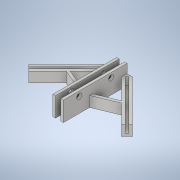
# Autodesk Inventor part: coffee
Saved by Autodesk Inventor 2021.1 (Build 251245010, 245A)
## iProperties
Created: 2019-12-05
Part Number: coffee
Material: Generic
Document SubType Name: Modeling
Designer: Christian
Density: 1 g/cm^3
Appearance: Default
Author: Christian
Autodesk Inventor part; units mm, degrees
ref_plane "YZ Plane" through (0, 0, 0) normal (1, 0, 0) x (0, 1, 0)
ref_plane "XZ Plane" through (0, 0, 0) normal (0, 1, 0) x (-1, 0, 0)
ref_plane "XY Plane" through (0, 0, 0) normal (0, 0, 1) x (1, 0, 0)
sketch "support_base" plane through (0, 0, 0) normal (0, 0, 1) x (1, 0, 0)
  line L0 (-24.7251, -5.2251) -> (20.2749, -5.2251)
  line L1 (20.2749, -5.2251) -> (20.2749, 0.7749)
  line L2 (20.2749, 0.7749) -> (-24.7251, 0.7749)
  line L3 (-24.7251, 0.7749) -> (-24.7251, -5.2251)
  line L4 (-24.7251, -5.2251) -> (20.2749, 0.7749) construction
  line L5 (20.2749, -5.2251) -> (-24.7251, 0.7749) construction
  line L6 (20.2749, 0.7749) -> (-11.5449, 32.5947)
  line L7 (-11.5449, 32.5947) -> (-10.1307, 34.009)
  line L8 (-10.1307, 34.009) -> (21.6892, 2.1892)
  line L9 (21.6892, 2.1892) -> (20.2749, 0.7749)
  line L10 (21.6892, 2.1892) -> (24.6892, -0.8108)
  line L11 (24.6892, -0.8108) -> (20.2749, -5.2251)
  line L12 (-2.2251, 0.7749) -> (4.365, 16.6848)
  line L13 (-4.3898, 0.7749) -> (2.8343, 18.2156)
  point P0 (4.5036, 7.635)
  point P1 (-2.2251, -2.2251)
  point P2 (-2.2251, -2.2251)
  dimension "d65" = 45
  dimension "d66" = 2
  dimension "d67" = 45
  dimension "d68" = 6
  dimension "d69" = 2
  measures "d65" angle of L2 L6
  measures "d66" distance of L6.end L7.end
  measures "d67" distance of L0.start L0.end
  measures "d68" distance of L2.end L0.start
  measures "d69" distance between parallel lines of L13 L12
sketch "Sketch11" plane through (0, 0, 0) normal (0, 0, 1) x (1, 0, 0)
  line L0 (0, 4) -> (0, -4) construction
  line L1 (2, 0) -> (0, 0) construction
  line L2 (40.0624, -5.0772) -> (8.2426, 26.7426)
  line L3 (8.2426, 26.7426) -> (4, 22.5)
  line L4 (4, 22.5) -> (35.8198, -9.3198)
  line L5 (35.8198, -9.3198) -> (40.0624, -5.0772)
  line L6 (40.0624, -5.0772) -> (4, 22.5) construction
  line L7 (8.2426, 26.7426) -> (35.8198, -9.3198) construction
  line L8 (4, 22.5) -> (4, -22.5)
  line L9 (4, -22.5) -> (2, -22.5)
  line L10 (2, -22.5) -> (2, 22.5)
  line L11 (2, 22.5) -> (4, 22.5)
  line L12 (2, 22.5) -> (2, 26.7426)
  line L13 (2, 26.7426) -> (8.2426, 26.7426)
  line L14 (19.9099, 6.5901) -> (4, 0)
  line L15 (21.4406, 5.0594) -> (4, -2.1648)
  line L16 (-40.0624, -5.0772) -> (-8.2426, 26.7426)
  line L17 (-8.2426, 26.7426) -> (-4, 22.5)
  line L18 (-4, 22.5) -> (-35.8198, -9.3198)
  line L19 (-35.8198, -9.3198) -> (-40.0624, -5.0772)
  line L20 (-40.0624, -5.0772) -> (-4, 22.5) construction
  line L21 (-8.2426, 26.7426) -> (-35.8198, -9.3198) construction
  line L22 (-4, 22.5) -> (-4, -22.5)
  line L23 (-4, -22.5) -> (-2, -22.5)
  line L24 (-2, -22.5) -> (-2, 22.5)
  line L25 (-2, 22.5) -> (-4, 22.5)
  line L26 (-2, 22.5) -> (-2, 26.7426)
  line L27 (-2, 26.7426) -> (-8.2426, 26.7426)
  line L28 (-19.9099, 6.5901) -> (-4, 0)
  line L29 (-21.4406, 5.0594) -> (-4, -2.1648)
  point P0 (2, 0)
  dimension "d80" = 2
  dimension "d81" = 8
  constraints: 4 end point, 3 vertical, 2 coincident, 1 horizontal, 1 midpoint, 1 other
  measures "d80" distance of L1.start L1.end
  measures "d81" distance of L0.start L0.end
extrude "Extrusion10" add sketch "Sketch11" along normal blind 8 contours L5 L4 L3 L2 | L3 L11 L12 L13 | L8 L9 L10 L11 | L15 L8 L14 L4 | L16 L17 L18 L19 | L27 L26 L25 L17 | L25 L24 L23 L22 | L18 L28 L22 L29
sketch "Sketch12" plane through (0, 0, 8) normal (0, 0, 1) x (1, 0, 0)
  line L0 (0, 28.3324) -> (0, -28.3324) construction
  line L1 (2, -22.5) -> (4, -22.5) construction
  line L2 (4, -22.5) -> (4, -2.1648) construction
  line L3 (4, -2.1648) -> (21.4406, 5.0594) construction
  line L4 (21.4406, 5.0594) -> (35.8198, -9.3198) construction
  line L5 (35.8198, -9.3198) -> (40.0624, -5.0772) construction
  line L6 (40.0624, -5.0772) -> (8.2426, 26.7426) construction
  line L7 (8.2426, 26.7426) -> (2, 26.7426) construction
  line L8 (2, 26.7426) -> (2, -22.5) construction
  line L9 (4, 22.5) -> (19.9099, 6.5901) construction
  line L10 (19.9099, 6.5901) -> (4, 0) construction
  line L11 (4, 0) -> (4, 22.5) construction
  line L12 (2, -22.5) -> (2, 26.7426)
  line L13 (2, 26.7426) -> (4, 26.7426)
  line L14 (4, 26.7426) -> (4, -22.5)
  line L15 (4, -22.5) -> (2, -22.5)
  line L16 (4, 0) -> (4, 22.5) projected
  line L17 (2, 26.7426) -> (2, -22.5) projected
  line L18 (2, -22.5) -> (4, -22.5) projected
  line L19 (8.2426, 26.7426) -> (2, 26.7426) projected
  line L20 (-2, -22.5) -> (-2, 26.7426)
  line L21 (-2, 26.7426) -> (-4, 26.7426)
  line L22 (-4, 26.7426) -> (-4, -22.5)
  line L23 (-4, -22.5) -> (-2, -22.5)
  line L24 (35.8198, -9.3198) -> (40.0624, -5.0772) projected
  line L25 (38.6482, -6.4914) -> (37.234, -7.9056)
  line L26 (37.234, -7.9056) -> (5.4142, 23.9142)
  line L27 (5.4142, 23.9142) -> (6.8284, 25.3284)
  line L28 (6.8284, 25.3284) -> (38.6482, -6.4914)
  line L29 (40.0624, -5.0772) -> (8.2426, 26.7426) projected
  line L30 (8.2426, 26.7426) -> (4, 22.5) construction
  line L31 (-38.6482, -6.4914) -> (-37.234, -7.9056)
  line L32 (-37.234, -7.9056) -> (-5.4142, 23.9142)
  line L33 (-5.4142, 23.9142) -> (-6.8284, 25.3284)
  line L34 (-6.8284, 25.3284) -> (-38.6482, -6.4914)
  point P0 (0, 0)
  point P1 (0, 0)
  point P2 (37.9411, -7.1985)
  dimension "d75" = 2
  constraints: 36 end point, 8 symmetric about line, 5 collinear, 4 parallel, 4 point on line, 3 midpoint, 2 coincident, 2 perpendicular, 1 vertical
  measures "d75" distance between parallel lines of L26 L28
extrude "Extrusion12" cut sketch "Sketch12" against normal blind 6 contours L26 L27 L28 L24 | L34 L33 L32 L31
extrude "Extrusion13" add sketch "Sketch12" along normal blind 15 from surface at -8 contours L12 L13 L14 L15 | L23 L22 L21 L20
sketch "Sketch13" plane through (4, 0, 0) normal (1, 0, 0) x (0, 0, -1)
  line L0 (-8, 26.7426) -> (-15, 26.7426) projected
  line L1 (0, -22.5) -> (-15, -22.5) projected
  line L2 (-15, 26.7426) -> (-15, -22.5) construction
  line L3 (-15, 2.1213) -> (-11.5, 2.1213) construction
  line L4 (-11.5, 2.1213) -> (-11.5, 26.7426) construction
  line L5 (-11.5, 2.1213) -> (-11.5, -22.5) construction
  point P0 (0, 0)
  point P1 (-11.5, 14.432)
  point P2 (-11.5, -10.1893)
  constraints: 6 end point, 4 midpoint, 2 point on line, 1 horizontal
hole "Hole1" at (4, 14.432, 11.5) at (4, -10.1893, 11.5) direction (-1, 0, 0) diameter 4 end through all
equation "\"d66\" = wall_t"
equation "\"d67\" = supp_h"
equation "\"d68\" = disp_t + 2 * wall_t"
equation "\"d69\" = wall_t"
equation "\"d80\" = wall_t"
equation "\"d81\" = 4 * wall_t"
equation "\"d70\" = disp_s + wall_t"
equation "\"d75\" = disp_t"
equation "\"d76\" = disp_s"
equation "\"d78\" = supp_b"
equation "\"d82\" = hole_d"
equation "\"wall_t\" = 2"
equation "\"disp_t\" = 2"
equation "\"supp_b\" = 15"
equation "\"disp_s\" = 6"
equation "\"supp_h\" = 45"
equation "\"hole_d\" = 4"
body "Solid4"
